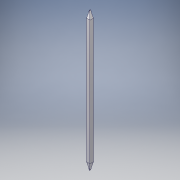
# Autodesk Inventor part: MM Support A
Saved by Autodesk Inventor 2018 (Build 220112000, 112)
## iProperties
Created: 2018-02-13
Part Number: MM Support A
Material: Iron, Malleable
Document SubType Name: Modeling
Designer: Marcus
Density: 7.15 g/cm^3
Appearance: Opal
Author: Marcus
Autodesk Inventor part; units mm, degrees
ref_plane "YZ Plane" through (0, 0, 0) normal (1, 0, 0) x (0, 1, 0)
sketch "Sketch5" plane through (0, 0, 0) normal (0, 1, 0) x (-1, 0, 0)
  line L0 (0, 0) -> (-914.4, 0)
  line L1 (-914.4, 0) -> (-914.4, -914.4)
  line L2 (-914.4, -914.4) -> (0, -914.4)
  line L3 (0, -914.4) -> (0, 0)
  dimension "d26" = 914.4
  dimension "d27" = 914.4
  constraints: 8 end point, 2 parallel, 1 horizontal, 1 perpendicular
  measures "d26" distance of L2.end L1.end
  measures "d27" distance of L1.end L0.end
extrude "Extrusion3" add sketch "Sketch5" along normal mid plane 33528
ref_plane "Work Plane4" through (0, 18288, 0) normal (0, 1, 0) x (1, 0, 0)
sketch "Sketch6" plane through (0, 18288, 0) normal (0, 1, 0) x (1, 0, 0)
  line L0 (609.6, 304.8) -> (304.8, 304.8)
  line L1 (304.8, 304.8) -> (304.8, 609.6)
  line L2 (304.8, 609.6) -> (609.6, 609.6)
  line L3 (609.6, 609.6) -> (609.6, 304.8)
  line L4 (914.4, 914.4) -> (0, 914.4) projected
  line L5 (914.4, 0) -> (914.4, 914.4) projected
  point P0 (0, 0)
  dimension "d31" = 304.8
  dimension "d32" = 304.8
  dimension "d33" = 304.8
  dimension "d34" = 304.8
  constraints: 8 end point, 2 parallel, 1 horizontal, 1 perpendicular
  measures "d31" distance of L1.end L2.end
  measures "d32" distance of L0.end L1.end
  measures "d33" distance between parallel lines of L4 L2
  measures "d34" distance between parallel lines of L5 L3
loft "Loft3" add profiles "Sketch6" section 1 edges at (457.2, 16764, 0) (914.4, 16764, -457.2) (457.2, 16764, -914.4) (0, 16764, -457.2)
ref_plane "Work Plane5" through (609.6, 18288, -304.8) normal (0, 0, -1) x (-1, 0, 0)
sketch "Sketch7" plane through (609.6, 18288, -304.8) normal (0, 0, -1) x (-1, 0, 0)
  line L0 (609.6, -1524) -> (304.8, 0) projected
  line L1 (0, 0) -> (304.8, 0) projected
  line L2 (-304.8, -1524) -> (0, 0) projected
  line L3 (304.8, 0) -> (0, 0) projected
  line L4 (304.8, 0) -> (240.3231, 322.3846)
  arc A0 (240.3231, 322.3846) -> (64.4769, 322.3846) centre (152.4, 304.8) ccw
  line L5 (-304.8, -1524) -> (0, 0) projected
  line L6 (64.4769, 322.3846) -> (0, 0)
  point P0 (609.6, -18288)
  dimension "d40" = 304.8
  constraints: 4 end point, 2 point on circle, 2 tangent, 1 centre point, 1 collinear, 1 equal length
  measures "d40" distance from line of L1 A0.centre
extrude "Extrusion4" add sketch "Sketch7" along normal up to surface (304.8 mm away)
hole "Hole1" at (457.2, 18592.8, -304.8) direction (0, 0, -1) diameter 76.2 end through all
mirror "Mirror1" about plane through (0, 0, 0) normal (0, 1, 0) of "Loft3", "Extrusion4", "Hole1"
ref_plane "Work Plane6" through (0, -18288, 0) normal (0, 1, 0) x (1, 0, 0)
ref_plane "Work Plane7" through (609.6, -18288, -304.8) normal (0, 0, 1) x (-1, 0, 0)
body "Solid2"
